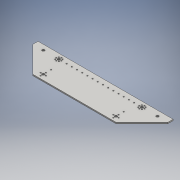
# Autodesk Inventor part: bot plate
Saved by Autodesk Inventor 2016 (Build 200138000, 138)
## iProperties
Created: 2016-01-25
Part Number: bot plate
Material: Generic
Document SubType Name: Modeling
Designer: TimB
Density: 1 g/cm^3
Appearance: Default
Author: TimB
Autodesk Inventor part; units mm, degrees
ref_plane "YZ Plane" through (0, 0, 0) normal (1, 0, 0) x (0, 1, 0)
ref_plane "XZ Plane" through (0, 0, 0) normal (0, 1, 0) x (-1, 0, 0)
ref_plane "XY Plane" through (0, 0, 0) normal (0, 0, 1) x (1, 0, 0)
sketch "Sketch1" plane through (0, 0, 0) normal (0, 0, 1) x (1, 0, 0)
  line L0 (-208, 48) -> (208, 48)
  line L1 (208, -48) -> (-208, 48) construction
  line L2 (-208, -48) -> (208, 48) construction
  circle A0 centre (176, 32) radius 4 projected
  circle A1 centre (-176, 32) radius 4 projected
  circle A2 centre (-128, 40) radius 1.85 projected
  circle A3 centre (-133.6569, 37.6569) radius 1.85 projected
  circle A4 centre (-136, 32) radius 1.85 projected
  circle A5 centre (-133.6569, 26.3431) radius 1.85 projected
  circle A6 centre (-128, 24) radius 1.85 projected
  circle A7 centre (-128, 32) radius 4 projected
  circle A8 centre (-122.3431, 26.3431) radius 1.85 projected
  circle A9 centre (-120, 32) radius 1.85 projected
  circle A10 centre (-122.3431, 37.6569) radius 1.85 projected
  circle A11 centre (128, 40) radius 1.85 projected
  circle A12 centre (122.3431, 37.6569) radius 1.85 projected
  circle A13 centre (120, 32) radius 1.85 projected
  circle A14 centre (122.3431, 26.3431) radius 1.85 projected
  circle A15 centre (128, 24) radius 1.85 projected
  circle A16 centre (133.6569, 26.3431) radius 1.85 projected
  circle A17 centre (128, 32) radius 4 projected
  circle A18 centre (136, 32) radius 1.85 projected
  circle A19 centre (133.6569, 37.6569) radius 1.85 projected
  circle A20 centre (104, 32) radius 1.85 projected
  circle A21 centre (88, 32) radius 1.85 projected
  circle A22 centre (72, 32) radius 1.85 projected
  circle A23 centre (56, 32) radius 1.85 projected
  circle A24 centre (40, 32) radius 1.85 projected
  circle A25 centre (24, 32) radius 1.85 projected
  circle A26 centre (8, 32) radius 1.85 projected
  circle A27 centre (-8, 32) radius 1.85 projected
  circle A28 centre (-24, 32) radius 1.85 projected
  circle A29 centre (-40, 32) radius 1.85 projected
  circle A30 centre (-56, 32) radius 1.85 projected
  circle A31 centre (-72, 32) radius 1.85 projected
  circle A32 centre (-88, 32) radius 1.85 projected
  circle A33 centre (-104, 32) radius 1.85 projected
  line L3 (-208, 48) -> (-208, 32)
  line L4 (-128, -48) -> (-208, 32)
  line L5 (208, 48) -> (208, 32)
  line L6 (128, -48) -> (208, 32)
  line L7 (128, -48) -> (-128, -48)
  point P0 (0, 0)
  dimension "d0" = 416
  dimension "d1" = 96
  dimension "d22" = 16
  dimension "d23" = 80
  dimension "d24" = 16
  constraints: 16 end point, 2 midpoint, 1 horizontal
  measures "d0" distance of L0.start L0.end
  measures "d1" distance of L2.start L0.start
  measures "d22" distance of L0.start L3.end
  measures "d23" distance of L2.start L4.start
  measures "d24" distance of L0.end L5.end
extrude "Extrusion2" add sketch "Sketch1" along normal blind 4
sketch "Sketch2" plane through (0, 0, 0) normal (0, 0, -1) x (-1, 0, 0)
  circle A0 centre (-112, -32) radius 4 projected
  circle A1 centre (112, -32) radius 4 projected
  point P0 (0, 0)
sketch "Sketch3" plane through (0, 0, 0) normal (0, 0, -1) x (-1, 0, 0)
  circle A0 centre (-112, -24) radius 1.85 projected
  circle A1 centre (-104, -32) radius 1.85 projected
  circle A2 centre (-112, -40) radius 1.85 projected
  circle A3 centre (-120, -32) radius 1.85 projected
  circle A4 centre (-112, -8) radius 1.85 projected
  circle A5 centre (112, -8) radius 1.85 projected
  circle A6 centre (120, -32) radius 1.85 projected
  circle A7 centre (112, -40) radius 1.85 projected
  circle A8 centre (104, -32) radius 1.85 projected
  circle A9 centre (112, -24) radius 1.85 projected
  point P0 (0, 0)
hole "Hole1" at (112, -32, 0) at (-112, -32, 0) direction (0, 0, 1) diameter 8 end through all
hole "Hole2" at (-112, -24, 0) at (-112, -8, 0) at (-120, -32, 0) at (-112, -40, 0) at (-104, -32, 0) at (112, -8, 0) at (120, -32, 0) at (112, -40, 0) at (104, -32, 0) at (112, -24, 0) direction (0, 0, 1) diameter 3.7 end through all
body "Solid2"
